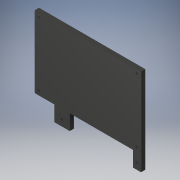
# Autodesk Inventor part: BA12
Saved by Autodesk Inventor 2017 (Build 210142000, 142)
## iProperties
Created: 2018-10-18
Part Number: BA12
Material: ABS Plastic
Document SubType Name: Modeling
Designer: Dell
Density: 1.06 g/cm^3
Appearance: Smooth - Black
Author: Dell
Autodesk Inventor part; units mm, degrees
ref_plane "YZ Plane" through (0, 0, 0) normal (1, 0, 0) x (0, 1, 0)
ref_plane "XZ Plane" through (0, 0, 0) normal (0, 1, 0) x (-1, 0, 0)
ref_plane "XY Plane" through (0, 0, 0) normal (0, 0, 1) x (1, 0, 0)
sketch "Sketch1" plane through (0, 0, 0) normal (0, 0, 1) x (1, 0, 0)
  line L0 (0, 0) -> (262.89, 0)
  line L1 (262.89, 0) -> (262.89, 177.8)
  line L2 (262.89, 177.8) -> (0, 177.8)
  line L3 (0, 177.8) -> (0, 0)
  dimension "d0" = 262.89
  dimension "d1" = 177.8
  constraints: 8 end point, 2 parallel, 1 horizontal, 1 perpendicular
  measures "d0" distance of L2.end L1.end
  measures "d1" distance of L1.end L0.end
extrude "Extrusion1" add sketch "Sketch1" along normal blind 10
sketch "Sketch3" plane through (0, 0, 10) normal (0, 0, 1) x (1, 0, 0)
  line L0 (0, 0) -> (262.89, 0) construction
  line L1 (262.89, 0) -> (262.89, 177.8) construction
  line L2 (262.89, 177.8) -> (0, 177.8) construction
  line L3 (0, 177.8) -> (0, 0) construction
  line L4 (10, 167.8) -> (252.89, 167.8) construction
  line L5 (252.89, 167.8) -> (252.89, 10) construction
  line L6 (252.89, 10) -> (10, 10) construction
  line L7 (10, 10) -> (10, 167.8) construction
  circle A0 centre (10, 167.8) radius 2.5
  circle A1 centre (10, 10) radius 2.5
  circle A2 centre (252.89, 10) radius 2.5
  circle A3 centre (252.89, 167.8) radius 2.5
  dimension "d4" = 10
  dimension "d5" = 5
  dimension "d6" = 5
  dimension "d7" = 5
  dimension "d8" = 5
  constraints: 8 end point, 4 centre point, 4 coincident, 3 other
  measures "d4" distance between parallel lines of L2 L4
  measures "d5" diameter of A0
  measures "d6" diameter of A1
  measures "d7" diameter of A2
  measures "d8" diameter of A3
extrude "Extrusion2" cut sketch "Sketch3" against normal through all
sketch "Sketch4" plane through (0, 0, 10) normal (0, 0, 1) x (1, 0, 0)
  line L0 (48.1, 0) -> (86.2, 0)
  line L1 (86.2, 0) -> (86.2, -38.1)
  line L2 (86.2, -38.1) -> (48.1, -38.1)
  line L3 (48.1, -38.1) -> (48.1, 0)
  line L4 (0, 177.8) -> (0, 0) projected
  line L5 (0, 0) -> (262.89, 0) projected
  line L6 (262.89, 0) -> (243.84, 0)
  line L7 (243.84, 0) -> (243.84, -38.1)
  line L8 (243.84, -38.1) -> (262.89, -38.1)
  line L9 (262.89, -38.1) -> (262.89, 0)
  circle A0 centre (67.15, -23.1) radius 2.5
  circle A1 centre (253.365, -23.1) radius 2.5
  point P0 (67.15, -38.1)
  point P1 (253.365, -38.1)
  dimension "d11" = 38.1
  dimension "d12" = 38.1
  dimension "d13" = 48.1
  dimension "d14" = 19.05
  dimension "d15" = 5
  dimension "d16" = 5
  dimension "d17" = 15
  constraints: 16 end point, 4 parallel, 2 centre point, 2 horizontal, 2 horizontal alignment, 2 midpoint, 2 perpendicular, 2 vertical alignment, 1 point on line
  measures "d11" distance of L1.end L2.end
  measures "d12" distance of L0.end L1.end
  measures "d13" distance between parallel lines of L3 L4
  measures "d14" distance of L7.end L8.end
  measures "d15" diameter of A0
  measures "d16" diameter of A1
  measures "d17" distance from line of L2 A0.centre
extrude "Extrusion3" add sketch "Sketch4" against normal blind 10
body "Solid1"
